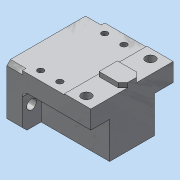
# Autodesk Inventor part: BC-10019-B
Saved by Autodesk Inventor 2016 (Build 200138000, 138)
## iProperties
Created: 2015-11-27
Part Number: BC-10019-B
Project: DIPOLO BC-3T- SIRIUS
Cost Center: 1504002005
Material: Alumínio 7075
Document SubType Name: Modeling
Designer: reinaldo.basilio
Mass: 1013.33 g
Surface Area: 413.826 cm^2
Volume: 360.616 cm^3
Density: 2.81 g/cm^3
Appearance: Anodized - White
Description: Fixador do polo de alto campo.
RuleStatus: InUse
AfterMaterialChange0: file://_iMaterial
AfterAnyiPropertyChange0: file://_iMaterial
AfterDocNew0: file://_Naming_par
AfterDocNew1: file://_NameStart
AfterDocNew2: file://_NameStart1
AfterDocNew3: file://_Materiais
DocNumber: XXXXX-XXX-XXXX-00-001.ipt
Folder: .
Title: DIPOLO BC-3T- SIRIUS
Author: reinaldo.basilio
Subject: BC-10019-B
Autodesk Inventor part; units mm, degrees
ref_plane "YZ Plane" through (0, 0, 0) normal (1, 0, 0) x (0, 1, 0)
ref_plane "XZ Plane" through (0, 0, 0) normal (0, 1, 0) x (-1, 0, 0)
ref_plane "XY Plane" through (0, 0, 0) normal (0, 0, 1) x (1, 0, 0)
sketch "Sketch5" plane through (0, 0, 0) normal (0, 1, 0) x (-1, 0, 0)
  line L0 (45, 30) -> (-45, 30)
  line L1 (-45, 30) -> (-45, -30)
  line L2 (-45, -30) -> (45, -30)
  line L3 (45, -30) -> (45, 30)
  point P0 (0, 0)
  point P1 (0, 30)
  point P2 (45, 0)
  dimension "d8" = 90
  dimension "d9" = 60
  constraints: 8 end point, 2 midpoint, 2 parallel, 1 horizontal, 1 horizontal alignment, 1 perpendicular, 1 vertical alignment
  measures "d8" distance of L0.start L0.end
  measures "d9" distance of L0.end L1.end
extrude "Extrusion5" add sketch "Sketch5" along normal blind 91.85
sketch "Sketch6" plane through (-45, 0, 30) normal (0, 0, 1) x (1, 0, 0)
  line L0 (0, 0) -> (90, 0) projected
  line L1 (0, 91.85) -> (90, 91.85) projected
  line L2 (35, 91.85) -> (55, 91.85)
  line L3 (55, 91.85) -> (55, 65.85)
  line L4 (55, 65.85) -> (35, 65.85)
  line L5 (35, 65.85) -> (35, 91.85)
  point P0 (45, 0)
  point P1 (45, 65.85)
  point P2 (45, 0)
  dimension "d12" = 26
  dimension "d13" = 20
  constraints: 8 end point, 2 midpoint, 2 parallel, 1 collinear, 1 horizontal, 1 perpendicular, 1 vertical alignment
  measures "d12" distance of L4.end L2.start
  measures "d13" distance of L3.end L4.end
extrude "Extrusion6" add sketch "Sketch6" along normal blind 5
chamfer "Chamfer2" distance 5 angle 45 2 edges at (10, 91.85, 32.5) (-10, 91.85, 32.5)
sketch "Sketch8" plane through (45, 0, -30) normal (0, 0, -1) x (-1, 0, 0)
  line L0 (0, 0) -> (90, 0) projected
  line L1 (90, 0) -> (90, 91.85) projected
  line L2 (0, 91.85) -> (90, 91.85) projected
  line L3 (0, 0) -> (0, 91.85) projected
  line L4 (20.5, 17) -> (20.5, 91.85)
  line L5 (45, 0) -> (45, 11.253)
  line L6 (45, 91.85) -> (45, 84.4514)
  line L7 (69.5, 91.85) -> (69.5, 17)
  line L8 (77.5, 17) -> (90, 17)
  line L9 (77.5, 17) -> (69.5, 17)
  line L10 (20.5, 17) -> (0, 17)
  point P0 (20.5, 25)
  point P1 (12.5, 17)
  point P2 (69.5, 25)
  dimension "d42" = 90
  constraints: 14 end point, 7 point on line, 4 vertical, 3 horizontal, 2 midpoint, 1 vertical alignment
  measures "d42" distance of L2.start L1.end
extrude "Extrusion7" cut sketch "Sketch8" against normal blind 40 contours L3 L2 L4 L10 | L8 L9 L7 L2 L1
sketch "Sketch9" plane through (45, 0, 10) normal (0, 0, -1) x (-1, 0, 0)
  circle A0 centre (10, 77) radius 5
  circle A1 centre (80, 77) radius 5
  line L0 (0, 0) -> (90, 0) projected
  line L1 (0, 17) -> (0, 91.85) projected
  circle A2 centre (10, 77) radius 10
  line L2 (0, 91.85) -> (90, 91.85)
  line L3 (45, 91.85) -> (45, 95.8754) construction
  line L4 (20.5, 91.85) -> (20.5, 17) construction
  point P0 (45, 0)
  dimension "d47" = 10
  dimension "d56" = 70
  dimension "d58" = 77
  dimension "d61" = 20
  dimension "d62" = 35
  dimension "d63" = 20.5
  constraints: 4 end point, 3 centre point, 1 coincident, 1 equal radius, 1 horizontal, 1 horizontal alignment, 1 midpoint, 1 vertical
  measures "d47" diameter of A0
  measures "d56" distance of A1.centre A0.centre
  measures "d58" distance from line of L0 A0.centre
  measures "d61" diameter of A2
  measures "d62" distance from line of L3 A0.centre
  measures "d63" distance between parallel lines of L1 L4
hole "Hole2" at (-35, 77, 10) at (35, 77, 10) direction (0, 0, 1) diameter 10.5 end through all
fillet "Fillet3" radius 6 2 edges at (34.75, 17, 10) (-34.75, 17, 10)
sketch "Sketch11" plane through (0, 0, 0) normal (0, -1, 0) x (1, 0, 0)
  line L0 (45, -30) -> (-45, -30) projected
  circle A0 centre (-35, -8) radius 5.25
  circle A1 centre (35, -8) radius 5.25
  circle A2 centre (-35, -8) radius 10
  line L1 (-24.5, 4) -> (-45, 4) projected
  point P0 (0, 0)
  dimension "d64" = 70
  dimension "d65" = 10.5
  dimension "d66" = 20
  dimension "d67" = 22
  dimension "d75" = 35
  dimension "d76" = 34
  constraints: 3 centre point, 1 coincident, 1 equal radius, 1 horizontal alignment
  measures "d64" distance of A1.centre A0.centre
  measures "d65" diameter of A0
  measures "d66" diameter of A2
  measures "d67" distance from line of A0.centre L0
  measures "d75" horizontal distance of point (0, 0) A0.centre
  measures "d76" distance between parallel lines of L0 L1
hole "Hole3" at (-35, 0, -8) at (35, 0, -8) direction (0, 1, 0) diameter 10.5 end through all
sketch "Sketch12" plane through (45, 0, 30) normal (1, 0, 0) x (0, 0, -1)
  line L0 (0, 0) -> (0, 91.85) projected
  line L1 (0, 0) -> (60, 0) projected
  line L2 (0, 0) -> (1, 0)
  line L3 (1, 0) -> (1, 63)
  line L4 (1, 63) -> (0, 63)
  line L5 (0, 63) -> (0, 0)
  point P0 (30, 0)
  dimension "d77" = 1
  dimension "d78" = 63
  dimension "d79" = 0
  constraints: 8 end point, 2 parallel, 1 collinear, 1 horizontal, 1 perpendicular
  measures "d77" distance between parallel lines of L3 L0
  measures "d78" distance of L2.end L3.end
  measures "d79" distance between parallel lines of L1 L2
extrude "Extrusion8" cut sketch "Sketch12" against normal through all
sketch "Sketch13" plane through (45, 0, 10) normal (0, 0, -1) x (-1, 0, 0)
  circle A0 centre (10, 77) radius 5.25 projected
  circle A1 centre (10, 48) radius 4
  circle A2 centre (10, 27) radius 4
  line L0 (0, 0) -> (90, 0) projected
  circle A3 centre (80, 77) radius 5.25 projected
  line L1 (45, 0) -> (45, -5.7212)
  circle A4 centre (80, 48) radius 4
  circle A5 centre (80, 27) radius 4
  dimension "d82" = 27
  dimension "d83" = 70
  dimension "d84" = 8
  dimension "d85" = 48
  constraints: 4 centre point, 2 end point, 2 symmetric about line, 2 vertical alignment, 1 equal radius, 1 vertical, 2 other
  measures "d82" distance from line of A2.centre L0
  measures "d83" distance of A3.centre A0.centre
  measures "d84" diameter of A2
  measures "d85" vertical distance of A1.centre L0.start
hole "Hole4" at (35, 48, 10) at (35, 27, 10) at (-35, 48, 10) at (-35, 27, 10) direction (0, 0, 1) diameter 6.647 end through all thread size "M8x1.25" class "6H" standard "ISO Metric profile"
sketch "Sketch16" plane through (0, 0, 0) normal (0, -1, 0) x (1, 0, 0)
  line L0 (-45, 29) -> (-41, 29)
  line L1 (-45, 25) -> (-45, 29)
  line L2 (-45, 25) -> (-41, 29)
  line L3 (0, 0) -> (0, -4.4881)
  line L4 (45, 29) -> (41, 29)
  line L5 (45, 25) -> (45, 29)
  line L6 (45, 25) -> (41, 29)
  line L7 (0, 0) -> (2.8094, 0)
  line L8 (-45, -30) -> (-40, -30)
  line L9 (-45, -25) -> (-45, -30)
  line L10 (-45, -25) -> (-40, -30)
  line L11 (45, -30) -> (40, -30)
  line L12 (45, -25) -> (45, -30)
  line L13 (45, -25) -> (40, -30)
  line L14 (45, -30) -> (-45, -30) projected
  line L15 (45, 29) -> (45, -30) projected
  dimension "d96" = 4
  dimension "d97" = 4
  dimension "d100" = 5
  dimension "d101" = 5
  dimension "d102" = 5
  dimension "d103" = 5
  dimension "d104" = 4
  constraints: 28 end point, 3 collinear, 2 horizontal, 2 symmetric about line, 1 vertical
  measures "d96" distance of L0.start L0.end
  measures "d97" distance of L1.start L0.start
  measures "d100" distance of L8.start L9.start
  measures "d101" distance of L8.start L8.end
  measures "d102" distance of L11.start L11.end
  measures "d103" distance of L12.start L11.start
  measures "d104" distance of L5.start L4.start
extrude "Extrusion10" cut sketch "Sketch16" against normal up to surface (17 mm away) from surface at 0
equation "\"d62\" = 0.5 * d56"
equation "\"d75\" = 0.5 * d64"
equation "\"d102\" = d101"
equation "\"d103\" = d100"
body "Solid5"
